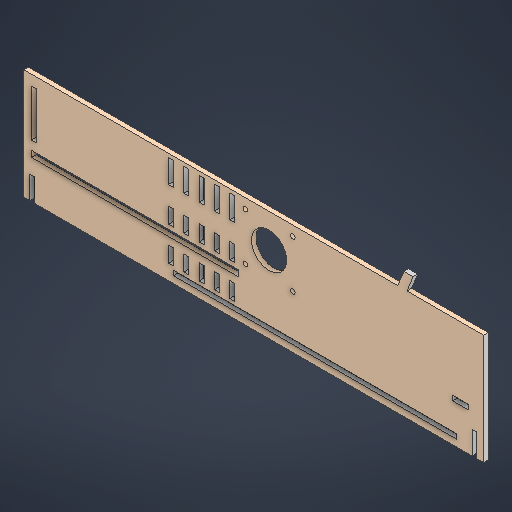
# Autodesk Inventor part: Sideboard
Saved by Autodesk Inventor 2027 (Build 310192000, 192)
## iProperties
Created: 2026-05-09
Part Number: Sideboard
Material: Generic
Document SubType Name: Modeling
Designer: alexy
Density: 1 g/cm^3
Appearance: Default
Author: alexy
Autodesk Inventor part; units mm, degrees
ref_plane "YZ Plane" through (0, 0, 0) normal (1, 0, 0) x (0, 1, 0)
ref_plane "XZ Plane" through (0, 0, 0) normal (0, 1, 0) x (-1, 0, 0)
ref_plane "XY Plane" through (0, 0, 0) normal (0, 0, 1) x (1, 0, 0)
sketch "Sketch1" plane through (0, 0, 0) normal (0, 0, 1) x (1, 0, 0)
  line L0 (0, 0) -> (300, 0)
  line L1 (300, 0) -> (300, 62)
  line L2 (300, 62) -> (0, 62)
  line L3 (0, 62) -> (0, 0)
  circle A0 centre (144.5, 55.5) radius 1.55
  circle A1 centre (144.5, 24.5) radius 1.55
  circle A2 centre (175.5, 55.5) radius 1.55
  circle A3 centre (175.5, 24.5) radius 1.55
  circle A4 centre (160, 40) radius 11.5
  line L4 (5, 19) -> (140, 19)
  line L5 (140, 19) -> (140, 15)
  line L6 (140, 15) -> (5, 15)
  line L7 (5, 15) -> (5, 19)
  line L8 (0, 62) -> (39.6145, 62)
  line L9 (8.1, 24.8) -> (5, 24.8)
  line L10 (5, 24.8) -> (5, 55.2)
  line L11 (5, 55.2) -> (8.1, 55.2)
  line L12 (8.1, 55.2) -> (8.1, 24.8)
  line L13 (8.1, 24.8) -> (5, 55.2) construction
  line L14 (5, 24.8) -> (8.1, 55.2) construction
  line L15 (0, 62) -> (50, 62)
  line L16 (0, 0) -> (0, -10)
  line L17 (0, -10) -> (300, -10)
  line L18 (300, -10) -> (300, 0)
  point P0 (6.55, 40)
  point P1 (5, 40)
  point P2 (8.1, 40)
  point P3 (5, 17)
  point P4 (140, 17)
  dimension "d1" = 3.1
  dimension "d2" = 3.1
  dimension "d3" = 3.1
  dimension "d4" = 3.1
  dimension "d5" = 31
  dimension "d7" = 23
  dimension "d8" = 15.5
  dimension "d9" = 15.5
  dimension "d10" = 62
  dimension "d11" = 31
  dimension "d13" = 40
  dimension "d54" = 300
  dimension "d55" = 3.1
  dimension "d56" = 5
  dimension "d57" = 15.2
  dimension "d59" = 135
  dimension "d93" = 15
  dimension "d106" = 20
  dimension "d107" = 5
  dimension "d201" = 4
  dimension "d202" = 10
  constraints: 38 end point, 6 midpoint, 6 parallel, 5 centre point, 5 perpendicular, 4 horizontal, 3 horizontal alignment, 2 vertical alignment, 1 vertical
  measures "d1" diameter of A0
  measures "d2" diameter of A1
  measures "d3" diameter of A2
  measures "d4" diameter of A3
  measures "d5" distance of A1.centre A3.centre
  measures "d7" diameter of A4
  measures "d8" horizontal distance of A0.centre A4.centre
  measures "d9" horizontal distance of A4.centre A3.centre
  measures "d10" distance of L0.end L1.end
  measures "d11" distance of A3.centre A2.centre
  measures "d13" distance from line of L0 A4.centre
  measures "d54" distance of L0.end L0.start
  measures "d55" distance of L10.end L11.end
  measures "d56" distance between parallel lines of L3 L10
  measures "d57" distance of point (5, 40) L10.end
  measures "d59" distance of L5.end L6.end
  measures "d93" distance between parallel lines of L0 L6
  measures "d106" horizontal distance of point (140, 17) A4.centre
  measures "d107" distance from line of L3 point (5, 17)
  measures "d201" distance of L6.end L4.start
  measures "d202" distance of L0.start L16.end
extrude "Extrusion1" add sketch "Sketch1" along normal blind 3
sketch "Sketch4" plane through (0, 0, 3) normal (0, 0, 1) x (1, 0, 0)
  line L0 (300, 62) -> (0, 62) projected
  line L1 (244, 62) -> (248, 72)
  line L2 (248, 72) -> (254, 72)
  line L3 (254, 72) -> (250, 62)
  line L4 (0, -10) -> (300, -10) projected
  point P0 (0, 0)
  dimension "d108" = 10
  dimension "d109" = 4
  dimension "d110" = 50
  dimension "d111" = 6
  constraints: 6 end point, 2 parallel, 2 point on line
  measures "d108" distance from line of L0 L1.end
  measures "d109" horizontal distance of L1.start L1.end
  measures "d110" distance of L0.start L3.end
  measures "d111" distance of L2.end L1.end
extrude "Extrusion4" add sketch "Sketch4" against normal blind 3
sketch "Sketch7" plane through (0, 0, 3) normal (0, 0, 1) x (1, 0, 0)
  line L0 (134.4, 59.6) -> (137.6, 59.6)
  line L1 (137.6, 59.6) -> (137.6, 44.4)
  line L2 (137.6, 44.4) -> (134.4, 44.4)
  line L3 (134.4, 44.4) -> (134.4, 59.6)
  line L4 (134.4, 59.6) -> (137.6, 44.4) construction
  line L5 (137.6, 59.6) -> (134.4, 44.4) construction
  line L6 (134.4, 32.1) -> (137.6, 32.1)
  line L7 (137.6, 32.1) -> (137.6, 21.9)
  line L8 (137.6, 21.9) -> (134.4, 21.9)
  line L9 (134.4, 21.9) -> (134.4, 32.1)
  line L10 (134.4, 32.1) -> (137.6, 21.9) construction
  line L11 (137.6, 32.1) -> (134.4, 21.9) construction
  line L12 (244, 62) -> (0, 62) projected
  circle A0 centre (144.5, 55.5) radius 1.55 projected
  line L13 (124.4, 59.6) -> (127.6, 59.6)
  line L14 (127.6, 59.6) -> (127.6, 44.4)
  line L15 (127.6, 44.4) -> (124.4, 44.4)
  line L16 (124.4, 44.4) -> (124.4, 59.6)
  line L17 (124.4, 59.6) -> (127.6, 44.4) construction
  line L18 (127.6, 59.6) -> (124.4, 44.4) construction
  line L19 (124.4, 32.1) -> (127.6, 32.1)
  line L20 (127.6, 32.1) -> (127.6, 21.9)
  line L21 (127.6, 21.9) -> (124.4, 21.9)
  line L22 (124.4, 21.9) -> (124.4, 32.1)
  line L23 (124.4, 32.1) -> (127.6, 21.9) construction
  line L24 (127.6, 32.1) -> (124.4, 21.9) construction
  line L25 (114.4, 59.6) -> (117.6, 59.6)
  line L26 (117.6, 59.6) -> (117.6, 44.4)
  line L27 (117.6, 44.4) -> (114.4, 44.4)
  line L28 (114.4, 44.4) -> (114.4, 59.6)
  line L29 (114.4, 59.6) -> (117.6, 44.4) construction
  line L30 (117.6, 59.6) -> (114.4, 44.4) construction
  line L31 (114.4, 32.1) -> (117.6, 32.1)
  line L32 (117.6, 32.1) -> (117.6, 21.9)
  line L33 (117.6, 21.9) -> (114.4, 21.9)
  line L34 (114.4, 21.9) -> (114.4, 32.1)
  line L35 (114.4, 32.1) -> (117.6, 21.9) construction
  line L36 (117.6, 32.1) -> (114.4, 21.9) construction
  line L37 (104.4, 59.6) -> (107.6, 59.6)
  line L38 (107.6, 59.6) -> (107.6, 44.4)
  line L39 (107.6, 44.4) -> (104.4, 44.4)
  line L40 (104.4, 44.4) -> (104.4, 59.6)
  line L41 (104.4, 59.6) -> (107.6, 44.4) construction
  line L42 (107.6, 59.6) -> (104.4, 44.4) construction
  line L43 (104.4, 32.1) -> (107.6, 32.1)
  line L44 (107.6, 32.1) -> (107.6, 21.9)
  line L45 (107.6, 21.9) -> (104.4, 21.9)
  line L46 (104.4, 21.9) -> (104.4, 32.1)
  line L47 (104.4, 32.1) -> (107.6, 21.9) construction
  line L48 (107.6, 32.1) -> (104.4, 21.9) construction
  line L49 (94.4, 59.6) -> (97.6, 59.6)
  line L50 (97.6, 59.6) -> (97.6, 44.4)
  line L51 (97.6, 44.4) -> (94.4, 44.4)
  line L52 (94.4, 44.4) -> (94.4, 59.6)
  line L53 (94.4, 59.6) -> (97.6, 44.4) construction
  line L54 (97.6, 59.6) -> (94.4, 44.4) construction
  line L55 (94.4, 32.1) -> (97.6, 32.1)
  line L56 (97.6, 32.1) -> (97.6, 21.9)
  line L57 (97.6, 21.9) -> (94.4, 21.9)
  line L58 (94.4, 21.9) -> (94.4, 32.1)
  line L59 (94.4, 32.1) -> (97.6, 21.9) construction
  line L60 (97.6, 32.1) -> (94.4, 21.9) construction
  line L61 (134.4, 10.1) -> (137.6, 10.1)
  line L62 (137.6, 10.1) -> (137.6, -0.1)
  line L63 (137.6, -0.1) -> (134.4, -0.1)
  line L64 (134.4, -0.1) -> (134.4, 10.1)
  line L65 (134.4, 10.1) -> (137.6, -0.1) construction
  line L66 (137.6, 10.1) -> (134.4, -0.1) construction
  line L67 (127.6, 10.1) -> (127.6, -0.1)
  line L68 (127.6, -0.1) -> (124.4, -0.1)
  line L69 (124.4, 10.1) -> (127.6, 10.1)
  line L70 (124.4, -0.1) -> (124.4, 10.1)
  line L71 (124.4, 10.1) -> (127.6, -0.1) construction
  line L72 (127.6, 10.1) -> (124.4, -0.1) construction
  line L73 (117.6, 10.1) -> (117.6, -0.1)
  line L74 (117.6, -0.1) -> (114.4, -0.1)
  line L75 (114.4, 10.1) -> (117.6, 10.1)
  line L76 (114.4, -0.1) -> (114.4, 10.1)
  line L77 (114.4, 10.1) -> (117.6, -0.1) construction
  line L78 (117.6, 10.1) -> (114.4, -0.1) construction
  line L79 (107.6, 10.1) -> (107.6, -0.1)
  line L80 (107.6, -0.1) -> (104.4, -0.1)
  line L81 (104.4, 10.1) -> (107.6, 10.1)
  line L82 (104.4, -0.1) -> (104.4, 10.1)
  line L83 (104.4, 10.1) -> (107.6, -0.1) construction
  line L84 (107.6, 10.1) -> (104.4, -0.1) construction
  line L85 (97.6, 10.1) -> (97.6, -0.1)
  line L86 (97.6, -0.1) -> (94.4, -0.1)
  line L87 (94.4, 10.1) -> (97.6, 10.1)
  line L88 (94.4, -0.1) -> (94.4, 10.1)
  line L89 (94.4, 10.1) -> (97.6, -0.1) construction
  line L90 (97.6, 10.1) -> (94.4, -0.1) construction
  line L91 (0, -10) -> (300, -10) projected
  line L92 (300, -10) -> (300, 62) projected
  point P0 (0, 0)
  point P1 (136, 52)
  point P2 (136, 27)
  point P3 (126, 52)
  point P4 (126, 27)
  point P5 (116, 52)
  point P6 (116, 27)
  point P7 (106, 52)
  point P8 (106, 27)
  point P9 (96, 52)
  point P10 (96, 27)
  point P11 (134.4, 52)
  point P12 (114.4, 52)
  point P13 (136, 5)
  point P14 (126, 5)
  point P15 (116, 5)
  point P16 (106, 5)
  point P17 (96, 5)
  point P18 (134.4, 5)
  point P19 (114.4, 5)
  point P20 (150, -10)
  dimension "d147" = 3.2
  dimension "d148" = 15.2
  dimension "d149" = 10.2
  dimension "d150" = 25
  dimension "d151" = 10
  dimension "d153" = 3.2
  dimension "d154" = 15.2
  dimension "d155" = 10.2
  dimension "d156" = 25
  dimension "d157" = 3.2
  dimension "d158" = 15.2
  dimension "d159" = 10.2
  dimension "d160" = 25
  dimension "d161" = 3.2
  dimension "d162" = 15.2
  dimension "d163" = 10.2
  dimension "d164" = 25
  dimension "d165" = 3.2
  dimension "d166" = 15.2
  dimension "d167" = 10.2
  dimension "d168" = 25
  dimension "d169" = 10
  dimension "d170" = 10
  dimension "d171" = 10
  dimension "d172" = 10
  dimension "d181" = 3.2
  dimension "d183" = 3.2
  dimension "d185" = 3.2
  dimension "d187" = 3.2
  dimension "d189" = 3.2
  dimension "d191" = 10
  dimension "d192" = 10
  dimension "d193" = 10
  dimension "d194" = 10
  dimension "d234" = 15
  dimension "d235" = 10.2
  dimension "d245" = 164
  constraints: 180 end point, 35 midpoint, 30 parallel, 15 horizontal, 15 perpendicular, 12 horizontal alignment, 6 vertical alignment, 5 point on line
  measures "d147" distance of L1.end L2.end
  measures "d148" distance of L2.end L0.start
  measures "d149" distance of L8.end L6.start
  measures "d150" distance of point (136, 27) point (136, 52)
  measures "d151" distance from line of L12 point (136, 52)
  measures "d153" distance of L14.end L15.end
  measures "d154" distance of L15.end L13.start
  measures "d155" distance of L22.start L19.start
  measures "d156" distance of point (126, 27) point (126, 52)
  measures "d157" distance of L26.end L27.end
  measures "d158" distance of L27.end L25.start
  measures "d159" distance of L34.start L31.start
  measures "d160" distance of point (116, 27) point (116, 52)
  measures "d161" distance of L38.end L39.end
  measures "d162" distance of L39.end L37.start
  measures "d163" distance of L46.start L43.start
  measures "d164" distance of point (106, 27) point (106, 52)
  measures "d165" distance of L50.end L51.end
  measures "d166" distance of L51.end L49.start
  measures "d167" distance of L58.start L55.start
  measures "d168" distance of point (96, 27) point (96, 52)
  measures "d169" distance of point (126, 52) point (136, 52)
  measures "d170" distance of point (126, 52) point (116, 52)
  measures "d171" distance of point (106, 52) point (116, 52)
  measures "d172" distance of point (96, 52) point (106, 52)
  measures "d181" distance of L63.start L63.end
  measures "d183" distance of L67.end L70.start
  measures "d185" distance of L73.end L78.end
  measures "d187" distance of L79.end L82.start
  measures "d189" distance of L85.end L86.end
  measures "d191" distance of point (126, 5) point (136, 5)
  measures "d192" distance of point (126, 5) point (116, 5)
  measures "d193" distance of point (106, 5) point (116, 5)
  measures "d194" distance of point (96, 5) point (106, 5)
  measures "d234" vertical distance of point (150, -10) point (136, 5)
  measures "d235" distance of L62.start L63.start
  measures "d245" distance from line of L92 point (136, 52)
extrude "Extrusion6" cut sketch "Sketch7" against normal blind 3 contours L0 L1 L2 L3 | L6 L7 L8 L9 | L13 L14 L15 L16 | L19 L20 L21 L22 | L25 L26 L27 L28 | L31 L32 L33 L34 | L37 L38 L39 L40 | L43 L44 L45 L46 | L49 L50 L51 L52 | L55 L56 L57 L58 | L61 L62 L63 L64 | L67 L68 L70 L69 | L73 L74 L76 L75 | L79 L80 L82 L81 | L85 L86 L88 L87
sketch "Sketch8" plane through (0, 0, 3) normal (0, 0, 1) x (1, 0, 0)
  line L0 (0, -10) -> (300, -10) projected
  line L1 (279.8, 18) -> (290, 18)
  line L2 (290, 18) -> (290, 14.8)
  line L3 (290, 14.8) -> (279.8, 14.8)
  line L4 (279.8, 14.8) -> (279.8, 18)
  line L5 (300, -10) -> (300, 62) projected
  line L6 (4, 5) -> (7.2, 5)
  line L7 (7.2, 5) -> (7.2, -10)
  line L8 (7.2, -10) -> (4, -10)
  line L9 (4, -10) -> (4, 5)
  line L10 (4, 5) -> (7.2, -10) construction
  line L11 (7.2, 5) -> (4, -10) construction
  line L12 (97.6, -2.45) -> (282.6, -2.45)
  line L13 (282.6, -2.45) -> (282.6, -5.55)
  line L14 (282.6, -5.55) -> (97.6, -5.55)
  line L15 (97.6, -5.55) -> (97.6, -2.45)
  line L16 (97.6, -2.45) -> (282.6, -5.55) construction
  line L17 (282.6, -2.45) -> (97.6, -5.55) construction
  line L18 (137.6, 10.1) -> (137.6, -0.1) projected
  line L19 (295.5, 5) -> (292.5, 5)
  line L20 (292.5, 5) -> (292.5, -10)
  line L21 (292.5, -10) -> (295.5, -10)
  line L22 (295.5, -10) -> (295.5, 5)
  line L23 (295.5, 5) -> (292.5, -10) construction
  line L24 (292.5, 5) -> (295.5, -10) construction
  point P0 (0, 0)
  point P1 (5.6, -2.5)
  point P2 (4, -2.5)
  point P3 (190.1, -4)
  point P4 (137.6, 5)
  point P5 (97.6, -0.1)
  point P6 (294, -2.5)
  dimension "d219" = 28
  dimension "d220" = 3.2
  dimension "d221" = 10.2
  dimension "d222" = 10
  dimension "d223" = 3.2
  dimension "d224" = 15
  dimension "d225" = 4
  dimension "d236" = 3.1
  dimension "d237" = 9
  dimension "d246" = 185
  dimension "d247" = 3
  dimension "d248" = 6
  dimension "d249" = 15
  constraints: 44 end point, 8 midpoint, 8 parallel, 4 horizontal, 4 perpendicular, 1 horizontal alignment, 1 point on line, 1 vertical alignment
  measures "d219" distance between parallel lines of L0 L1
  measures "d220" distance of L3.end L1.start
  measures "d221" distance of L2.end L3.end
  measures "d222" distance between parallel lines of L5 L2
  measures "d223" distance of L7.end L8.end
  measures "d224" distance of L6.end L7.end
  measures "d225" distance of L0.start L8.end
  measures "d236" distance of L14.end L12.start
  measures "d237" vertical distance of point (190.1, -4) point (137.6, 5)
  measures "d246" distance of L13.end L14.end
  measures "d247" distance between parallel lines of L20 L22
  measures "d248" distance from line of L5 point (294, -2.5)
  measures "d249" distance of L21.end L19.start
extrude "Extrusion7" cut sketch "Sketch8" against normal blind 3
body "Solid1"
